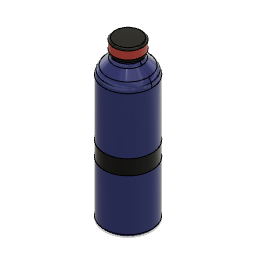
FOOBO v4 (Autodesk Fusion 360 design; units mm, degrees)
Autodesk Fusion 360 part; units mm, degrees
sketch "Schizzo1" plane through (0, 0, 0) normal (0, 0, 1) x (1, 0, 0) in component "Bottle"
  line L0 (0, 0) -> (40, 0)
  line L1 (40, 0) -> (40, 90)
  line L2 (40, 90) -> (20, 110)
  line L3 (20, 110) -> (20, 130)
  line L4 (20, 130) -> (0, 130)
  line L5 (0, -2) -> (42, -2)
  line L6 (42, -2) -> (42, 90.8284)
  line L7 (42, 90.8284) -> (22, 110.8284)
  line L8 (22, 110.8284) -> (22, 132)
  line L9 (22, 132) -> (0, 132)
  line L10 (0, 132) -> (0, 130)
  line L11 (0, 0) -> (0, -2)
  line L12 (42, -2) -> (42, -17)
  line L13 (40.0289, -2) -> (40.0289, -17)
  line L14 (40.0289, -17) -> (42, -17)
  dimension "d1" = 90
  dimension "d2" = 2
  dimension "d3" = 15
  constraint coincident L0.start L11.start
  constraint horizontal L0
  constraint perpendicular L0 L1
  constraint parallel L1 L3
  constraint perpendicular L3 L4
  constraint perpendicular L4 L10
  constraint perpendicular L5 L12
  constraint coincident L5 L13.start
  constraint perpendicular L5 L13
  measures "d1" distance of L0.end L1.end
  measures "d3" distance of L5.end L12.end
revolve "Rivoluzione1" add sketch "Schizzo1" angle 360 about axis through (0, 1.75, 0) along (0, 1, 0) makes body 1 in component "Bottle"
fillet "Raccordo1" chord length 15 1 edges at (-39.1577, 90.8284, -15.1878) on bodies 1 in component "Bottle"
fillet "Raccordo2" chord length 6 1 edges at (-20.5112, 110.8284, -7.9555) on bodies 1 in component "Bottle"
sketch "Schizzo2" plane through (0, 132, 0) normal (0, 1, 0) x (-1, 0, 0) in component "Bottle"
  circle A0 centre (0, 0) radius 22
  circle A1 centre (0, 0) radius 20
  constraint coincident A0.centre A1.centre
extrude "Estrudi1" cut sketch "Schizzo2" against normal blind 5 contours A1 bodies 1 in component "Bottle"
sketch "Schizzo1 (2)" plane through (0, 132, 0) normal (0, 1, 0) x (-1, 0, 0) in component "tappo"
  circle A0 centre (0, 0) radius 20
  circle A1 centre (0, 0) radius 22
  circle A2 centre (0, 0) radius 20
  circle A3 centre (0, 0) radius 23
  circle A4 centre (0, 0) radius 25
  dimension "d12" = 46
  dimension "d13" = 50
  constraint concentric A0 A2
  constraint concentric A0 A3
  constraint concentric A2 A4
  measures "d12" diameter of A3
  measures "d13" diameter of A4
extrude "Estrudi2" add sketch "Schizzo1 (2)" against normal blind 15 separate body contours A0 A2 makes body 2 in component "tappo"
extrude "Estrudi1'" add sketch "Schizzo1 (2)" along normal blind 7 separate body contours A0 A2 | A1 | A3 | A4 makes body 3 in component "tappo"
extrude "Estrudi3" add sketch "Schizzo1 (2)" against normal blind 15 contours A4 bodies 3 in component "tappo"
fillet "Raccordo1'" radius 3 1 edges at (23.3082, 139, -9.0404) on bodies 3 in component "tappo"
fillet "Raccordo2'" radius 7.5 1 edges at (23.3082, 117, 9.0404) on bodies 3 in component "tappo"
sketch "Schizzo1 (3)" plane through (0, -17, 0) normal (0, -1, 0) x (1, 0, 0) in component "separatore"
  circle A0 centre (0, 0) radius 42
  circle A1 centre (0, 0) radius 40.0289
  circle A2 centre (0, 0) radius 42
  circle A3 centre (0, 0) radius 40.0289
  circle A4 centre (0, 0) radius 37.5
  dimension "d22" = 75
  constraint coincident A0.centre A1.centre
  constraint concentric A2 A4
  measures "d22" diameter of A4
extrude "Estrudi2'" add sketch "Schizzo1 (3)" along normal blind 8 separate body contours A0 A2 | A1 A3 | A4 makes body 4 in component "separatore"
extrude "Estrudi1''" add sketch "Schizzo1 (3)" against normal blind 13 separate body contours A1 A3 makes body 5 in component "separatore"
sketch "Schizzo2 (2)" plane through (0, -25, 0) normal (0, -1, 0) x (1, 0, 0) in component "separatore"
  circle A0 centre (0, 0) radius 42
  circle A1 centre (0, 0) radius 42
  circle A2 centre (0, 0) radius 40
  constraint coincident A0.centre A1.centre
  constraint concentric A1 A2
extrude "Estrudi3'" add sketch "Schizzo2 (2)" along normal blind 18 bodies 4 in component "separatore"
sketch "Schizzo1 (4)" plane through (0, -43, 0) normal (0, -1, 0) x (1, 0, 0) in component "food box"
  circle A0 centre (0, 0) radius 40
  circle A1 centre (0, 0) radius 42
  circle A2 centre (0, 0) radius 37.5
  circle A3 centre (0, 0) radius 40
  circle A4 centre (0, 0) radius 42
  circle A5 centre (0, 0) radius 42
  dimension "d29" = 75
  constraint concentric A0 A2
  constraint concentric A2 A3
  constraint concentric A3 A4
  constraint concentric A4 A5
  measures "d29" diameter of A2
extrude "Estrudi2''" add sketch "Schizzo1 (4)" along normal blind 85 separate body contours A0 A3 | A1 A4 A5 makes body 6 in component "food box"
extrude "Estrudi1'''" add sketch "Schizzo1 (4)" against normal blind 15 separate body contours A0 A3 makes body 7 in component "food box"
sketch "Schizzo3" plane through (0, -128, 0) normal (0, -1, 0) x (1, 0, 0) in component "food box"
  circle A0 centre (0, 0) radius 37.5
  circle A1 centre (0, 0) radius 42
  circle A2 centre (0, 0) radius 37.5
  constraint concentric A0 A2
extrude "Estrudi3''" add sketch "Schizzo3" along normal blind 10 separate body contours A0 A2 makes body 8 in component "food box"
extrude "Estrudi4" add 1 faces at (40.204, -128, -3.9496) along direction (0, -1, 0) blind 10 on bodies 6 bodies 6 8 in component "food box"
fillet "Raccordo1''" radius 5 1 edges at (-39.1577, -138, -15.1878) on bodies 6 in component "food box"
component "Bottle" placed x (1, 0, 0) y (0, 1, 0) z (0, 0, 1) at (0, 0, 0)
component "tappo" placed x (1, 0, 0) y (0, 1, 0) z (0, 0, 1) at (0, 0, 0)
component "separatore" placed x (1, 0, 0) y (0, 1, 0) z (0, 0, 1) at (0, 0, 0)
component "food box" placed x (1, 0, 0) y (0, 1, 0) z (0, 0, 1) at (0, 0, 0)
